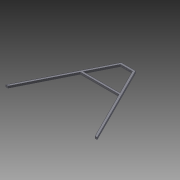
# Autodesk Inventor part: CAVALETE_SUPERIOR
Saved by Autodesk Inventor 2015 (Build 190159000, 159)
## iProperties
Manager: Standard
Created: 2016-02-21
Part Number: CAVALETE_SUPERIOR
Material: SAE 1010/1020
Document SubType Name: Modeling
Designer: Everton
Authority: Rafael Salvador
Manufacturer: Standard
Standards Organization: Custom
Density: 7.86 g/cm^3
Appearance: Steel
Author: Everton
Comments: -
Revision Number: 00
Autodesk Inventor part; units mm, degrees
ref_plane "YZ Plane" through (0, 0, 0) normal (1, 0, 0) x (0, 1, 0)
ref_plane "XZ Plane" through (0, 0, 0) normal (0, 1, 0) x (-1, 0, 0)
ref_plane "XY Plane" through (0, 0, 0) normal (0, 0, 1) x (1, 0, 0)
sketch "Sketch1" plane through (0, 0, 0) normal (0, 0, 1) x (1, 0, 0)
  line L0 (9.7407, 1114.2593) -> (159.7407, 1114.2593)
  line L1 (9.7407, 1114.2593) -> (-140.2593, 1114.2593)
  line L2 (-943.4843, -492.1907) -> (-140.2593, 1114.2593)
  line L3 (159.7407, 1114.2593) -> (962.9657, -492.1907)
  line L4 (918.2444, -492.1907) -> (135.0194, 1074.2593)
  line L5 (135.0194, 1074.2593) -> (9.7407, 1074.2593)
  line L6 (9.7407, 1074.2593) -> (-115.5379, 1074.2593)
  line L7 (-115.5379, 1074.2593) -> (-898.7629, -492.1907)
  line L8 (9.7407, 554.2593) -> (395.0194, 554.2593)
  line L9 (9.7407, 554.2593) -> (-375.5379, 554.2593)
  line L10 (415.0194, 514.2593) -> (9.7407, 514.2593)
  line L11 (9.7407, 514.2593) -> (-395.5379, 514.2593)
  line L12 (-635.5379, 34.2593) -> (-680.2593, 34.2593)
  line L13 (9.7407, 34.2593) -> (9.7407, -477.7407)
  line L14 (-785.5379, -265.7407) -> (-830.2593, -265.7407)
  line L15 (-830.2593, -265.7407) -> (-785.5379, -265.7407)
  line L16 (911.0194, -477.7407) -> (955.7407, -477.7407)
  line L17 (955.7407, -477.7407) -> (911.0194, -477.7407)
  line L18 (-891.5379, -477.7407) -> (-936.2593, -477.7407)
  line L19 (918.2444, -492.1907) -> (962.9657, -492.1907)
  line L20 (-943.4843, -492.1907) -> (-898.7629, -492.1907)
  point P0 (0, 0)
  point P1 (655.0194, 34.2593)
  point P2 (699.7407, 34.2593)
  point P3 (-670.2593, 54.2593)
  dimension "d4" = 40
  dimension "d5" = 40
  dimension "d12" = 40
  dimension "d23" = 512
  constraints: 42 end point, 16 point on line, 5 horizontal, 1 perpendicular, 1 vertical
  measures "d4" distance between parallel lines of L3 L4
  measures "d5" distance between parallel lines of L2 L7
  measures "d12" distance between parallel lines of L8 L10
  measures "d23" distance of L13.start L13.end
extrude "Extrusion1" add sketch "Sketch1" along normal blind 40 contours L0 L3 L16 L4 L5 L6 L7 L12 L2 L1
fillet "Fillet1" radius 0.5 7 edges at (-245.5379, 814.2593, 40) (-515.5379, 274.2593, 40) (72.3801, 1074.2593, 40) (265.0194, 814.2593, 40) (557.7407, 318.2593, 40) (-65.2593, 1114.2593, 40) (-410.2593, 574.2593, 40)
fillet "Fillet2" radius 0.5 7 edges at (-410.2593, 574.2593, 0) (-245.5379, 814.2593, 0) (-515.5379, 274.2593, 0) (72.3801, 1074.2593, 0) (84.7407, 1114.2593, 0) (557.7407, 318.2593, 0) (265.0194, 814.2593, 0)
extrude "Extrusion2" add sketch "Sketch1" along normal blind 40 contours L10 L11 L7 L9 L8 L4
fillet "Fillet3" radius 0.5 3 edges at (9.7407, 554.2593, 0) (212.3801, 514.2593, 0) (212.3801, 514.2593, 40)
fillet "Fillet4" radius 0.5 1 edges at (9.7407, 554.2593, 40)
sketch "Sketch2" plane through (-140.2593, 1114.2593, 39.5) normal (0, 1, 0) x (1, 0, 0)
  line L0 (298.84, 0.606) -> (0.309, 39.5)
  line L1 (299.691, 39.5) -> (0, 0)
  circle A0 centre (150.8669, 19.8846) radius 2.5
  point P0 (140.2593, 39.5)
  dimension "d17" = 5
  constraints: 4 end point, 2 point on line, 1 centre point
  measures "d17" diameter of A0
extrude "Extrusion3" cut sketch "Sketch2" against normal blind 50
sketch "Sketch3" plane through (-140.2593, 1114.2593, 39.5) normal (0, 1, 0) x (1, 0, 0)
  point P0 (140.2593, 39.5)
sketch "Sketch4" plane through (-140.2593, 1114.2593, 39.5) normal (0, 1, 0) x (1, 0, 0)
  line L0 (226.7669, 24.5) -> (200.9669, 24.5) projected
  line L1 (226.7669, 24.5) -> (200.9669, 24.5) projected
  line L2 (200.9669, 14.5) -> (226.7669, 14.5) projected
  arc A0 (226.7669, 14.5) -> (226.7669, 24.5) centre (226.7669, 19.5) ccw projected
  arc A1 (200.9669, 24.5) -> (200.9669, 14.5) centre (200.9669, 19.5) ccw projected
  arc A2 (100.7669, 14.5) -> (100.7669, 24.5) centre (100.7669, 19.5) ccw projected
  line L3 (100.7669, 24.5) -> (74.9669, 24.5) projected
  line L4 (100.7669, 14.5) -> (74.9669, 14.5) projected
  arc A3 (74.9669, 24.5) -> (74.9669, 14.5) centre (74.9669, 19.5) ccw projected
  point P0 (140.2593, 39.5)
extrude "Extrusion4" cut sketch "Sketch4" against normal blind 50
extrude "Extrusion5" add sketch "Sketch1" along normal blind 40 contours L0 L3 L16 L4 L5 L6 L7 L12 L2 L1
extrude "Extrusion6" add sketch "Sketch1" along normal blind 40 contours L12 L7 L14 L2
extrude "Extrusion7" add sketch "Sketch1" along normal blind 40 contours L14 L7 L18 L2
extrude "Extrusion8" add sketch "Sketch1" along normal blind 40 contours L18 L7 L20 L2
extrude "Extrusion9" add sketch "Sketch1" along normal blind 40 contours L3 L19 L4 L16
sketch "Sketch5" plane through (-140.2593, 1114.2593, 0) normal (0, 1, 0) x (1, 0, 0)
  line L0 (535.5286, 0) -> (-235.5286, 0) projected
  line L1 (0.065, 0) -> (300, -40)
  line L2 (300, -40) -> (300, 0)
  line L3 (300, 0) -> (300, -40) projected
  line L4 (300, 0) -> (0.065, -40)
  circle A0 centre (150.0325, -20) radius 5
  point P0 (140.2593, 0)
  dimension "d38" = 10
  constraints: 6 end point, 1 centre point, 1 collinear, 1 midpoint, 1 point on line
  measures "d38" diameter of A0
extrude "Extrusion10" cut sketch "Sketch5" against normal blind 40 contours A0 L1 L4 | L4 L1 A0 | L1 L4 A0 | A0 L4 L1
sketch "Sketch6" plane through (-140.2593, 1114.2593, 0) normal (0, 1, 0) x (1, 0, 0)
  line L0 (225.9325, -25) -> (200.1325, -25) projected
  arc A0 (225.9325, -25) -> (225.9325, -15) centre (225.9325, -20) ccw projected
  line L1 (200.1325, -15) -> (225.9325, -15) projected
  arc A1 (200.1325, -15) -> (200.1325, -25) centre (200.1325, -20) ccw projected
  arc A2 (99.9325, -25) -> (99.9325, -15) centre (99.9325, -20) ccw projected
  line L2 (99.9325, -25) -> (74.1325, -25) projected
  arc A3 (74.1325, -15) -> (74.1325, -25) centre (74.1325, -20) ccw projected
  line L3 (74.1325, -15) -> (99.9325, -15) projected
  point P0 (140.2593, 0)
extrude "Extrusion11" cut sketch "Sketch6" against normal blind 50
body "Solid1"
